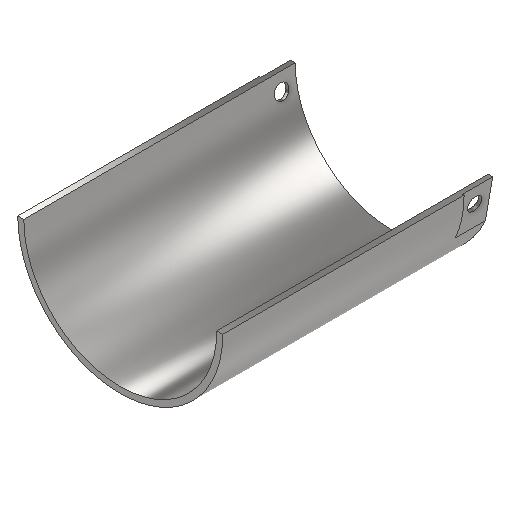
# Autodesk Inventor part: B_shield_5
Saved by Autodesk Inventor 2026.2 (Build 302298000, 298)
## iProperties
Created: 2026-02-20
Part Number: B_shield_5
Material: ステンレス鋼 440C
Document SubType Name: Modeling
Designer: zetsu
Density: 7.75 g/cm^3
Appearance: 半つや出し
Author: zetsu
Autodesk Inventor part; units mm, degrees
ref_plane "XZ Plane" through (0, 0, 0) normal (0, 1, 0) x (-1, 0, 0)
sketch "スケッチ1" plane through (0, 0, 0) normal (0, 0, 1) x (1, 0, 0)
  arc A0 (-17, 0) -> (17, 0) centre (0, 0) ccw
  arc A1 (-16, 0) -> (16, 0) centre (0, 0) ccw
  line L0 (-16, 0) -> (-17, 0)
  line L1 (16, 0) -> (17, 0)
  dimension "d0" = 17
  dimension "d66" = 1
  constraints: 6 point on circle, 4 end point, 3 line through centre, 2 centre point, 2 coincident
  measures "d0" radius of A0
  measures "d66" distance of L1.end L1.start
extrude "押し出し1" add sketch "スケッチ1" along normal blind 45
ref_plane "作業平面4" through (16.7417, -2.952, 0) normal (0.9848, -0.1736, 0) x (0, 0, 1)
ref_plane "作業平面3" through (0, 0, 0) normal (0.9848, -0.1736, 0) x (0, 0, 1)
ref_plane "作業平面6" through (-16.7417, -2.952, 0) normal (0.9848, 0.1736, 0) x (0, 0, 1)
ref_plane "作業平面5" through (0, 0, 0) normal (0.9848, 0.1736, 0) x (0, 0, 1)
sketch "スケッチ8" plane through (16.7417, -2.952, 0) normal (0.9848, -0.1736, 0) x (0, 0, 1)
  line L0 (0, -5) -> (5, -5)
  line L1 (5, -5) -> (5, 5)
  line L2 (5, 5) -> (0, 5)
  line L3 (0, 5) -> (0, -5)
  line L4 (0, 0) -> (8.4852, 0) construction
  dimension "d38" = 5
  dimension "d39" = 10
  constraints: 10 end point, 3 perpendicular, 2 horizontal, 1 other
  measures "d38" distance of L2.end L1.end
  measures "d39" distance of L1.end L0.end
extrude "押し出し8" cut sketch "スケッチ8" against normal blind 0.5
sketch "スケッチ9" plane through (-16.7417, -2.952, 0) normal (0.9848, 0.1736, 0) x (0, 0, 1)
  line L0 (0, -5) -> (5, -5)
  line L1 (5, -5) -> (5, 5)
  line L2 (5, 5) -> (0, 5)
  line L3 (0, 5) -> (0, -5)
  line L4 (0, 0) -> (8.3316, 0) construction
  dimension "d42" = 5
  dimension "d43" = 10
  constraints: 10 end point, 2 horizontal, 2 parallel, 1 perpendicular, 1 other
  measures "d42" distance of L1.end L2.end
  measures "d43" distance of L0.end L1.end
extrude "押し出し9" cut sketch "スケッチ9" along normal blind 0.5
sketch "スケッチ11" plane through (16.2493, -2.8652, 0) normal (0.9848, -0.1736, 0) x (0, 0, -1)
  circle A0 centre (-2.5, 0) radius 1.2
  point P0 (0, 0)
  dimension "d50" = 2.4
  dimension "d51" = 2.5
  constraints: 1 centre point
  measures "d50" diameter of A0
  measures "d51" distance of point (0, 0) A0.centre
extrude "押し出し11" cut sketch "スケッチ11" against normal blind 1
sketch "スケッチ12" plane through (-16.2493, -2.8652, 0) normal (-0.9848, -0.1736, 0) x (0, 0, 1)
  circle A0 centre (2.5, 0) radius 1.2
  point P0 (0, 0)
  dimension "d54" = 2.4
  dimension "d55" = 2.5
  constraints: 1 centre point
  measures "d54" diameter of A0
  measures "d55" distance of point (0, 0) A0.centre
extrude "押し出し12" cut sketch "スケッチ12" against normal blind 1
